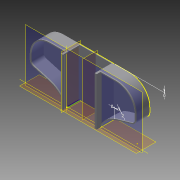
# Autodesk Inventor part: kontroller3
Saved by Autodesk Inventor 2015 (Build 190159000, 159)
## iProperties
Created: 2015-12-13
Part Number: kontroller3
Material: Generic
Document SubType Name: Modeling
Designer: abberik
Density: 1 g/cm^3
Appearance: Default
Author: abberik
Autodesk Inventor part; units mm, degrees
sketch "Sketch1" plane through (0, 0, 0) normal (0, 0, 1) x (1, 0, 0)
  line L0 (0, 0) -> (0, 24)
  line L1 (0, 24) -> (2, 24)
  line L2 (2, 24) -> (66, 24)
  line L3 (66, 24) -> (68, 24)
  line L4 (68, 24) -> (68, 0)
  line L5 (68, 0) -> (66, 0)
  line L6 (0, 0) -> (2, 0)
  line L7 (2, 0) -> (2, -2)
  line L8 (2, -2) -> (0, -2)
  line L9 (66, 0) -> (66, -2)
  line L10 (66, -2) -> (68, -2)
  line L11 (68, -2) -> (70, -2)
  line L12 (70, -2) -> (70, 24)
  line L13 (70, 24) -> (70, 26)
  line L14 (70, 26) -> (0, 26)
  line L15 (0, 26) -> (-2, 26)
  line L16 (-2, 26) -> (-2, -2)
  line L17 (-2, -2) -> (0, -2)
  dimension "d0" = 24
  dimension "d1" = 2
  dimension "d2" = 64
  dimension "d3" = 2
  dimension "d4" = 24
  dimension "d5" = 2
  dimension "d6" = 2
  dimension "d7" = 2
  dimension "d8" = 2
  dimension "d9" = 2
  dimension "d10" = 2
  constraints: 36 end point, 10 perpendicular, 5 point on line, 2 horizontal, 2 vertical
  measures "d0" distance of L0.start L0.end
  measures "d1" distance of L0.end L1.end
  measures "d2" distance of L1.end L2.end
  measures "d3" distance of L2.end L3.end
  measures "d4" distance of L3.end L4.end
  measures "d5" distance of L0.start L6.end
  measures "d6" distance of L6.end L7.end
  measures "d7" distance of L5.end L9.end
  measures "d8" distance of L10.end L11.end
  measures "d9" distance of L12.end L13.end
  measures "d10" distance of L14.end L15.end
extrude "Extrusion1" add sketch "Sketch1" along normal blind 96.5
sketch "Sketch2" plane through (0, 0, 0) normal (0, 0, -1) x (-1, 0, 0)
  line L0 (0, 0) -> (0, 24) projected
  line L1 (-2, 0) -> (0, 0) projected
  line L2 (-2, -2) -> (-2, 0) projected
  line L3 (2, -2) -> (-2, -2) projected
  line L4 (2, 26) -> (2, -2) projected
  line L5 (-70, 26) -> (2, 26) projected
  line L6 (-70, -2) -> (-70, 26) projected
  line L7 (-66, -2) -> (-70, -2) projected
  line L8 (-66, 0) -> (-66, -2) projected
  line L9 (-68, 0) -> (-66, 0) projected
  line L10 (-68, 24) -> (-68, 0) projected
  line L11 (0, 24) -> (-68, 24) projected
  line L12 (0, 24) -> (-68, 24) projected
  line L13 (-68, 0) -> (-66, 0)
  line L14 (-66, 0) -> (-66, 24)
  line L15 (-66, 24) -> (-68, 24)
  line L16 (-68, 24) -> (-68, 0)
  line L17 (0, 0) -> (-2, 0)
  line L18 (-2, 0) -> (-2, 24)
  line L19 (-2, 24) -> (0, 24)
  line L20 (0, 24) -> (0, 0)
  constraints: 16 end point, 4 parallel, 2 horizontal, 2 perpendicular, 2 point on line
sketch "Sketch5" plane through (-2, 26, 0) normal (0, 1, 0) x (1, 0, 0)
  line L0 (72, -96.5) -> (102.7802, -96.5)
  line L1 (142.7802, -56.5) -> (142.7802, -46.7352)
  line L2 (72, 0) -> (72, -96.5)
  arc A0 (102.7802, -96.5) -> (142.7802, -56.5) centre (102.7802, -56.5) ccw
  line L3 (72, 0) -> (72, -37.5452)
  line L4 (72, 0) -> (72, -96.5) projected
  line L5 (135.5549, -37.1279) -> (103.3741, -27.8337)
  arc A1 (72, 0) -> (104.5, -28.1589) centre (117.8095, 20.0371) ccw
  arc A2 (142.7802, -46.7352) -> (135.5549, -37.1279) centre (132.7802, -46.7352) ccw
  point P0 (2, 0)
  dimension "d18" = 40
  dimension "d20" = 50
  dimension "d21" = 10
  constraints: 10 end point, 7 point on circle, 4 tangent, 3 centre point, 2 point on line, 1 horizontal, 1 parallel, 1 perpendicular
  measures "d18" radius of A0
  measures "d20" radius of A1
  measures "d21" radius of A2
extrude "Extrusion3" add sketch "Sketch5" against normal up to surface (28 mm away) contours L2 A1 L5 A2 L1 A0 L0
sketch "Sketch6" plane through (-2, 26, 96.5) normal (0, 1, 0) x (1, 0, 0)
  line L0 (72, 96.5) -> (0, 96.5) projected
  line L1 (0, 96.5) -> (0, 0) projected
  line L2 (0, 0) -> (102.7802, 0) projected
  arc A0 (102.7802, 0) -> (142.7802, 40) centre (102.7802, 40) ccw projected
  line L3 (142.7802, 40) -> (142.7802, 49.7648) projected
  arc A1 (142.7802, 49.7648) -> (135.5549, 59.3721) centre (132.7802, 49.7648) ccw projected
  line L4 (135.5549, 59.3721) -> (104.5, 68.3411) projected
  arc A2 (72, 96.5) -> (104.5, 68.3411) centre (117.8095, 116.5371) ccw projected
  line L5 (70, 96.5) -> (70, 0) projected
  line L6 (70, 96.5) -> (70, 0) projected
  line L7 (70, 96.5) -> (70, 0) projected
  line L8 (72, 0) -> (72, 96.5)
  line L9 (103.9562, 66.4164) -> (135, 57.4507)
  arc A3 (140.7802, 49.7648) -> (135, 57.4507) centre (132.7802, 49.7648) ccw
  line L10 (140.7802, 49.7648) -> (140.7802, 40)
  arc A4 (102.7802, 2) -> (140.7802, 40) centre (102.7802, 40) ccw
  line L11 (102.7802, 2) -> (2, 2)
  line L12 (2, 2) -> (2, 94.5)
  line L13 (2, 94.5) -> (70.71, 94.5)
  arc A5 (70.71, 94.5) -> (103.9562, 66.4164) centre (117.8095, 116.5371) ccw
  line L14 (72, 91.9305) -> (72, 2)
  point P0 (2, 96.5)
  point P1 (70, 94.5)
  dimension "d24" = 0
  dimension "d25" = 0
  dimension "d26" = 2
  constraints: 14 end point, 7 point on circle, 3 centre point, 3 point on line, 1 parallel, 1 vertical, 7 other
  measures "d24" distance of L0.start L8.end
  measures "d25" distance from line of L2 L8.start
  measures "d26" radial gap between concentric circles of A2 A5
extrude "Extrusion4" cut sketch "Sketch6" against normal up to surface (28 mm away) contours A5 L9 A3 L10 A4 L11 L8
extrude "Extrusion5" add sketch "Sketch6" against normal blind 2 contours A5 L9 A3 L10 A4 L11 L8
ref_plane "Work Plane1" through (34, 0, 96.5) normal (-1, 0, 0) x (0, 0, 1)
mirror "Mirror1" about plane through (34, 0, 96.5) normal (-1, 0, 0) of "Extrusion4"
mirror "Mirror2" about plane through (34, 0, 96.5) normal (-1, 0, 0) of "Extrusion5", "Extrusion4", "Extrusion3"
sketch "Sketch8" plane through (0, 0, 96.5) normal (0, 0, 1) x (1, 0, 0)
  line L0 (0, 0) -> (0, 24) projected
  line L1 (0, 24) -> (68, 24) projected
  line L2 (68, 24) -> (68, 0) projected
  line L3 (68, 0) -> (66, 0) projected
  line L4 (66, 0) -> (66, -2) projected
  line L5 (66, -2) -> (100.7802, -2) projected
  line L6 (100.7802, 26) -> (100.7802, -2) projected
  line L7 (-32.7802, 26) -> (100.7802, 26) projected
  line L8 (-32.7802, 26) -> (-32.7802, -2) projected
  line L9 (2, -2) -> (-32.7802, -2) projected
  line L10 (2, -2) -> (2, 0) projected
  line L11 (2, 0) -> (0, 0) projected
  line L12 (0, 24) -> (2, 24)
  line L13 (2, 24) -> (2, 0)
  line L14 (2, 0) -> (0, 0)
  line L15 (0, 0) -> (0, 24)
  line L16 (68, 0) -> (66, 0)
  line L17 (66, 0) -> (66, 24)
  line L18 (66, 24) -> (68, 24)
  line L19 (68, 24) -> (68, 0)
  constraints: 16 end point, 4 parallel, 2 horizontal, 2 perpendicular, 1 point on line
extrude "Extrusion6" add sketch "Sketch8" against normal blind 2 contours L0 L1 L13 L11 | L1 L2 L3 L17
sketch "Sketch9" plane through (0, 0, 0) normal (0, 0, -1) x (-1, 0, 0)
  line L0 (-68, 0) -> (-66, 0) projected
  line L1 (-66, -2.009) -> (-68, -2.009)
  line L2 (-68, -2.009) -> (-68, 0)
  line L3 (-68, 0) -> (-66, 0)
  line L4 (-66, 0) -> (-66, -2.009)
  line L5 (-34, 31.6018) -> (-34, -7.6109) projected
  line L6 (0, 0) -> (-2, 0)
  line L7 (-2, -2.009) -> (0, -2.009)
  line L8 (0, -2.009) -> (0, 0)
  line L9 (-2, 0) -> (-2, -2.009)
  constraints: 16 end point, 5 symmetric about line, 2 parallel, 1 horizontal, 1 perpendicular
extrude "Extrusion7" cut sketch "Sketch9" against normal up to surface (94.5 mm away) contours L0 L4 L1 L2
mirror "Mirror3" about plane through (34, 0, 96.5) normal (-1, 0, 0) of "Extrusion7"
sketch "Sketch10" plane through (0, 0, 0) normal (0, 0, -1) x (-1, 0, 0)
  point P0 (0, 0)
sketch "Sketch11" plane through (0, 0, 0) normal (0, 0, -1) x (-1, 0, 0)
  line L0 (-68, -2) -> (-68, -4)
  line L1 (-68, -4) -> (-66, -4)
  line L2 (-66, -4) -> (-66, -6)
  line L3 (-66, -6) -> (-70, -6)
  line L4 (-70, -6) -> (-70, -2)
  line L5 (-70, -2) -> (-68, -2)
  point P0 (0, 0)
  dimension "d35" = 2
  dimension "d36" = 2
  dimension "d37" = 2
  dimension "d38" = 4
  constraints: 12 end point, 3 perpendicular, 1 horizontal, 1 vertical
  measures "d35" distance of L0.start L0.end
  measures "d36" distance of L0.end L1.end
  measures "d37" distance of L1.end L2.end
  measures "d38" distance of L2.end L3.end
sketch "Sketch12" plane through (66, -2, 96.5) normal (0, -1, 0) x (1, 0, 0)
  line L0 (0, -2) -> (4, -2) projected
  line L1 (0, -96.5) -> (0, -2) projected
  line L2 (0, -96.5) -> (4, -96.5) projected
  line L3 (4, -96.5) -> (4, -2) projected
  line L4 (4, -2) -> (34.7802, -2) projected
  arc A0 (72.7802, -40) -> (34.7802, -2) centre (34.7802, -40) ccw projected
  line L5 (72.7802, -40) -> (72.7802, -49.7648) projected
  arc A1 (67, -57.4507) -> (72.7802, -49.7648) centre (64.7802, -49.7648) ccw projected
  line L6 (67, -57.4507) -> (35.9562, -66.4164) projected
  arc A2 (35.9562, -66.4164) -> (4, -91.9305) centre (49.8095, -116.5371) ccw projected
  line L7 (4, -91.9305) -> (4, -2) projected
  arc A3 (36.5, -68.3411) -> (4, -96.5) centre (49.8095, -116.5371) ccw projected
  line L8 (67.5549, -59.3721) -> (36.5, -68.3411) projected
  arc A4 (67.5549, -59.3721) -> (74.7802, -49.7648) centre (64.7802, -49.7648) ccw projected
  line L9 (74.7802, -40) -> (74.7802, -49.7648) projected
  arc A5 (74.7802, -40) -> (34.7802, 0) centre (34.7802, -40) ccw projected
  line L10 (0, 0) -> (34.7802, 0) projected
  line L11 (0, -2) -> (0, 0) projected
  line L12 (0, -2) -> (2, -2) projected
  line L13 (4, -96.5) -> (4, -2) projected
  line L14 (4, -2) -> (0, -2)
  line L15 (0, -2) -> (0, 0)
  line L16 (0, 0) -> (4, 0)
  line L17 (4, 0) -> (4, -2)
  line L18 (2, -2) -> (2, -96.5) projected
  line L19 (2, -96.5) -> (4, -96.5) projected
  point P0 (-66, -96.5)
  constraints: 8 end point, 2 parallel, 1 horizontal, 1 perpendicular
extrude "Extrusion10" add sketch "Sketch11" against normal up to surface (94.5 mm away)
extrude "Extrusion11" add sketch "Sketch12" along normal up to surface (4 mm away) contours L11 L10 L17 L0
mirror "Mirror5" about plane through (34, 0, 96.5) normal (-1, 0, 0) of "Extrusion10"
mirror "Mirror6" about plane through (34, 0, 96.5) normal (-1, 0, 0) of "Extrusion10"
sketch "Sketch13" plane through (-32.7802, -2, 96.5) normal (0, -1, 0) x (1, 0, 0)
  line L0 (34.7802, -2) -> (30.7802, -2) projected
  line L1 (30.7802, -96.5) -> (30.7802, -2) projected
  line L2 (34.7802, -96.5) -> (30.7802, -96.5) projected
  line L3 (34.7802, -96.5) -> (34.7802, -2) projected
  line L4 (30.7802, -96.5) -> (30.7802, -91.9305) projected
  arc A0 (30.7802, -91.9305) -> (-1.176, -66.4164) centre (-15.0293, -116.5371) ccw projected
  line L5 (-1.176, -66.4164) -> (-32.2198, -57.4507) projected
  arc A1 (-38, -49.7648) -> (-32.2198, -57.4507) centre (-30, -49.7648) ccw projected
  line L6 (-38, -49.7648) -> (-38, -40) projected
  arc A2 (0, -2) -> (-38, -40) centre (0, -40) ccw projected
  line L7 (0, -2) -> (30.7802, -2) projected
  line L8 (30.7802, -2) -> (32.7802, -2) projected
  line L9 (32.7802, -2) -> (34.7802, -2) projected
  line L10 (34.7802, -2) -> (34.7802, 0) projected
  line L11 (34.7802, 0) -> (0, 0) projected
  arc A3 (0, 0) -> (-40, -40) centre (0, -40) ccw projected
  line L12 (-40, -40) -> (-40, -49.7648) projected
  arc A4 (-40, -49.7648) -> (-32.7747, -59.3721) centre (-30, -49.7648) ccw projected
  line L13 (-32.7747, -59.3721) -> (-1.7198, -68.3411) projected
  arc A5 (30.7802, -96.5) -> (-1.7198, -68.3411) centre (-15.0293, -116.5371) ccw projected
  line L14 (0, 0) -> (133.5605, 0) projected
  line L15 (34.7802, -2) -> (30.7802, -2)
  line L16 (30.7802, -2) -> (30.7802, 0)
  line L17 (30.7802, 0) -> (34.7802, 0)
  line L18 (34.7802, 0) -> (34.7802, -2)
  point P0 (32.7802, -96.5)
  constraints: 8 end point, 2 parallel, 1 horizontal, 1 perpendicular, 1 point on line
extrude "Extrusion12" add sketch "Sketch13" along normal up to surface (4 mm away) contours L0 L16 L11 L10
sketch "Sketch14" plane through (0, 0, 0) normal (0, 0, -1) x (-1, 0, 0)
  line L0 (2, 26) -> (2, -2) projected
  line L1 (-70, 26) -> (2, 26) projected
  line L2 (-70, -2) -> (-70, 26) projected
  line L3 (-70, -6) -> (-70, -2) projected
  line L4 (-66, -6) -> (-70, -6) projected
  line L5 (-66, -4) -> (-66, -6) projected
  line L6 (-68, -4) -> (-66, -4) projected
  line L7 (-68, 24) -> (-68, -4) projected
  line L8 (0, 24) -> (-68, 24) projected
  line L9 (0, -4) -> (0, 24) projected
  line L10 (0, -4) -> (-2, -4) projected
  line L11 (-2, -4) -> (-2, -6) projected
  line L12 (-2, -6) -> (2, -6) projected
  line L13 (2, -6) -> (2, -2) projected
  line L14 (-66, -6) -> (-70, -6) projected
  line L15 (-68, -6) -> (-68, -8)
  line L16 (-68, -8) -> (-66, -8)
  line L17 (-66, -8) -> (-66, -10)
  line L18 (-66, -10) -> (-70, -10)
  line L19 (-70, -10) -> (-70, -6)
  line L20 (-68, -6) -> (-70, -6)
  line L21 (-34, 33.6) -> (-34, -19.6) projected
  line L22 (0, -6) -> (0, -8)
  line L23 (0, -8) -> (-2, -8)
  line L24 (-2, -8) -> (-2, -10)
  line L25 (-2, -10) -> (2, -10)
  line L26 (2, -10) -> (2, -6)
  line L27 (0, -6) -> (2, -6)
  line L28 (-2, -6) -> (2, -6) projected
  point P0 (0, 0)
  dimension "d49" = 2
  dimension "d50" = 2
  dimension "d51" = 2
  dimension "d52" = 4
  constraints: 24 end point, 5 symmetric about line, 3 perpendicular, 2 collinear, 1 midpoint, 1 vertical
  measures "d49" distance of L15.start L15.end
  measures "d50" distance of L15.end L16.end
  measures "d51" distance of L16.end L17.end
  measures "d52" distance of L17.end L18.end
extrude "Extrusion13" add sketch "Sketch14" against normal up to surface (94.5 mm away) contours L26 L25 L24 L23 L22 L12 | L4 L15 L16 L17 L18 L19
sketch "Sketch15" plane through (-2, -6, 96.5) normal (0, -1, 0) x (1, 0, 0)
  line L0 (0, -2) -> (4, -2)
  line L1 (4, -2) -> (4, 0)
  line L2 (4, 0) -> (0, 0)
  line L3 (0, 0) -> (0, -2)
  point P0 (2, -96.5)
  constraints: 8 end point, 2 parallel, 1 horizontal, 1 perpendicular
extrude "Extrusion14" add sketch "Sketch15" along normal up to surface (4 mm away)
sketch "Sketch16" plane through (66, -6, 96.5) normal (0, -1, 0) x (1, 0, 0)
  line L0 (0, 0) -> (4, 0)
  line L1 (4, 0) -> (4, -2)
  line L2 (4, -2) -> (0, -2)
  line L3 (0, -2) -> (0, 0)
  point P0 (-66, -96.5)
  constraints: 8 end point, 2 parallel, 1 horizontal, 1 perpendicular
extrude "Extrusion15" add sketch "Sketch16" along normal up to surface (4 mm away)
ref_plane "Work Plane2" through (34, 0, 96.5) normal (-1, 0, 0) x (0, 0, 1)
body "Solid1"
